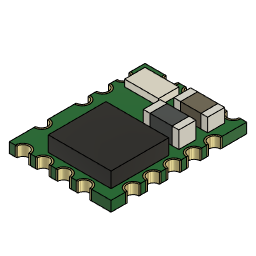
BLE-RN4871U v1 (Autodesk Fusion 360 design; units mm, degrees)
Autodesk Fusion 360 part; units mm, degrees
sketch "Sketch1" plane through (0, 0, 0) normal (0, 0, 1) x (1, 0, 0)
  arc A0 (6, 6.55) -> (6, 5.65) centre (6, 6.1) ccw
  arc A1 (6, 6.45) -> (6, 5.75) centre (6, 6.1) ccw
  arc A2 (6, 5.35) -> (6, 4.45) centre (6, 4.9) ccw
  arc A3 (6, 5.25) -> (6, 4.55) centre (6, 4.9) ccw
  arc A4 (6, 4.15) -> (6, 3.25) centre (6, 3.7) ccw
  arc A5 (6, 4.05) -> (6, 3.35) centre (6, 3.7) ccw
  arc A6 (6, 2.85) -> (6, 2.15) centre (6, 2.5) ccw
  arc A7 (6, 2.95) -> (6, 2.05) centre (6, 2.5) ccw
  arc A8 (6, 1.75) -> (6, 0.85) centre (6, 1.3) ccw
  arc A9 (6, 1.65) -> (6, 0.95) centre (6, 1.3) ccw
  arc A10 (4.85, 0) -> (3.95, 0) centre (4.4, 0) ccw
  arc A11 (4.75, 0) -> (4.05, 0) centre (4.4, 0) ccw
  arc A12 (3.65, 0) -> (2.75, 0) centre (3.2, 0) ccw
  arc A13 (3.55, 0) -> (2.85, 0) centre (3.2, 0) ccw
  arc A14 (2.45, 0) -> (1.55, 0) centre (2, 0) ccw
  arc A15 (2.35, 0) -> (1.65, 0) centre (2, 0) ccw
  arc A16 (1.25, 0) -> (0.35, 0) centre (0.8, 0) ccw
  arc A17 (1.15, 0) -> (0.45, 0) centre (0.8, 0) ccw
  arc A18 (0, 1.45) -> (0, 2.35) centre (0, 1.9) ccw
  arc A19 (0, 1.55) -> (0, 2.25) centre (0, 1.9) ccw
  arc A20 (0, 3.85) -> (0, 4.75) centre (0, 4.3) ccw
  arc A21 (0, 3.95) -> (0, 4.65) centre (0, 4.3) ccw
  arc A22 (0, 5.05) -> (0, 5.95) centre (0, 5.5) ccw
  arc A23 (0, 5.15) -> (0, 5.85) centre (0, 5.5) ccw
  arc A24 (0, 6.25) -> (0, 7.15) centre (0, 6.7) ccw
  arc A25 (0, 6.35) -> (0, 7.05) centre (0, 6.7) ccw
  arc A26 (1.15, 8) -> (2.05, 8) centre (1.6, 8) ccw
  arc A27 (1.25, 8) -> (1.95, 8) centre (1.6, 8) ccw
  arc A28 (2.35, 8) -> (3.25, 8) centre (2.8, 8) ccw
  arc A29 (2.45, 8) -> (3.15, 8) centre (2.8, 8) ccw
  arc A30 (3.65, 8) -> (4.35, 8) centre (4, 8) ccw
  arc A31 (3.55, 8) -> (4.45, 8) centre (4, 8) ccw
  arc A32 (4.75, 8) -> (5.65, 8) centre (5.2, 8) ccw
  arc A33 (4.85, 8) -> (5.55, 8) centre (5.2, 8) ccw
  line L0 (0, 1.55) -> (0, 0)
  line L1 (0, 3.95) -> (0, 2.25)
  line L2 (0, 5.15) -> (0, 4.65)
  line L3 (0, 8) -> (0, 7.05)
  line L4 (0, 6.35) -> (0, 5.85)
  line L5 (1.25, 8) -> (0, 8)
  line L6 (2.45, 8) -> (1.95, 8)
  line L7 (3.65, 8) -> (3.15, 8)
  line L8 (6, 8) -> (5.55, 8)
  line L9 (4.85, 8) -> (4.35, 8)
  line L10 (6, 6.45) -> (6, 8)
  line L11 (6, 5.25) -> (6, 5.75)
  line L12 (6, 4.05) -> (6, 4.55)
  line L13 (0, 0) -> (0.45, 0)
  line L14 (1.15, 0) -> (1.65, 0)
  line L15 (2.35, 0) -> (2.85, 0)
  line L16 (3.55, 0) -> (3.95, 0)
  line L17 (4.75, 0) -> (6, 0)
  line L18 (6, 0) -> (6, 0.95)
  line L19 (6, 1.65) -> (6, 2.15)
  line L20 (6, 2.85) -> (6, 3.35)
  line L21 (1.7, 4) -> (5.4, 4)
  line L22 (5.4, 4) -> (5.4, 0.6)
  line L23 (5.4, 0.6) -> (1.7, 0.6)
  line L24 (1.7, 0.6) -> (1.7, 4)
  line L25 (4.05, 0) -> (3.95, 0)
  line L26 (0.6, 7.4) -> (2.6, 7.4)
  line L27 (2.6, 7.4) -> (2.6, 6.2)
  line L28 (2.6, 6.2) -> (0.6, 6.2)
  line L29 (0.6, 6.2) -> (0.6, 7.4)
  line L30 (5.4, 4.6) -> (3.3, 4.6)
  line L31 (3.3, 4.6) -> (3.3, 5.6)
  line L32 (3.3, 5.6) -> (5.4, 5.6)
  line L33 (5.4, 5.6) -> (5.4, 4.6)
  line L34 (5.4, 6.3) -> (3.4, 6.3)
  line L35 (3.4, 6.3) -> (3.4, 7.3)
  line L36 (3.4, 7.3) -> (5.4, 7.3)
  line L37 (5.4, 7.3) -> (5.4, 6.3)
  line L38 (3.8, 6.3) -> (3.8, 7.3)
  line L39 (5, 6.3) -> (5, 7.3)
  line L40 (3.7, 5.6) -> (3.7, 4.6)
  line L41 (5, 5.6) -> (5, 4.6)
  constraint horizontal L13
  constraint vertical L18
  constraint horizontal L8
  constraint vertical L3
  constraint coincident L0.end L13.start
  constraint concentric A16 A17
  constraint concentric A14 A15
  constraint concentric A12 A13
  constraint concentric A10 A11
  constraint concentric A18 A19
  constraint concentric A20 A21
  constraint concentric A22 A23
  constraint concentric A24 A25
  constraint concentric A8 A9
  constraint concentric A6 A7
  constraint concentric A4 A5
  constraint concentric A2 A3
  constraint concentric A0 A1
  constraint concentric A26 A27
  constraint concentric A28 A29
  constraint concentric A30 A31
  constraint concentric A32 A33
  constraint coincident A0.end L18
  constraint coincident A0.start L18
  constraint coincident A1.start L18
  constraint coincident A2.end L18
  constraint coincident A2.start L18
  constraint coincident A3.start L18
  constraint coincident A4.end L18
  constraint coincident A4.start L18
  constraint coincident A5.start L18
  constraint coincident A6.end L18
  constraint coincident A6.start L18
  constraint coincident A7.end L18
  constraint coincident A7.start L18
  constraint coincident A8.end L18
  constraint coincident A8.start L18
  constraint coincident A9.start L18
  constraint coincident A10.end L13
  constraint coincident A10.start L13
  constraint coincident A11.end L13
  constraint coincident A11.start L13
  constraint coincident A12.end L13
  constraint coincident A12.start L13
  constraint coincident A13.end L13
  constraint coincident A13.start L13
  constraint coincident A14.end L13
  constraint coincident A14.start L13
  constraint coincident A15.end L13
  constraint coincident A15.start L13
  constraint coincident A16.end L13
  constraint coincident A16.start L13
  constraint coincident A17.start L13
  constraint coincident A18.end L3
  constraint coincident A18.start L3
  constraint coincident A19.start L3
  constraint coincident A20.end L3
  constraint coincident A20.start L3
  constraint coincident A21.start L3
  constraint coincident A22.end L3
  constraint coincident A22.start L3
  constraint coincident A23.start L3
  constraint coincident A24.end L3
  constraint coincident A24.start L3
  constraint coincident A25.start L3
  constraint coincident A26.end L8
  constraint coincident A26.start L8
  constraint coincident A27.start L8
  constraint coincident A28.end L8
  constraint coincident A28.start L8
  constraint coincident A29.start L8
  constraint coincident A30.start L8
  constraint coincident A31.end L8
  constraint coincident A31.start L8
  constraint coincident A32.end L8
  constraint coincident A32.start L8
  constraint coincident A33.start L8
  constraint collinear L0 L3
  constraint collinear L1 L3
  constraint collinear L2 L3
  constraint collinear L3 L4
  constraint collinear L5 L8
  constraint collinear L6 L8
  constraint collinear L7 L8
  constraint collinear L8 L9
  constraint collinear L10 L18
  constraint collinear L11 L18
  constraint collinear L12 L18
  constraint collinear L13 L14
  constraint collinear L14 L15
  constraint collinear L15 L16
  constraint collinear L16 L17
  constraint collinear L18 L19
  constraint collinear L19 L20
  constraint horizontal L21
  constraint vertical L22
  constraint horizontal L23
  constraint vertical L24
  constraint horizontal L26
  constraint vertical L27
  constraint horizontal L28
  constraint vertical L29
  constraint horizontal L32
  constraint vertical L33
  constraint horizontal L30
  constraint vertical L31
  constraint horizontal L36
  constraint vertical L37
  constraint horizontal L34
  constraint vertical L35
  constraint coincident L36 L38.end
  constraint perpendicular L36 L38
  constraint coincident L36 L39.end
  constraint perpendicular L36 L39
  constraint coincident L30 L40.end
  constraint perpendicular L30 L40
  constraint coincident L30 L41.end
  constraint perpendicular L30 L41
  constraint coincident L32 L40.start
  constraint coincident L34 L38.start
  constraint coincident L34 L39.start
  constraint coincident L32 L41.start
extrude "Extrude1" add sketch "Sketch1" along normal blind 0.6 contours A0 A2 A4 A7 A8 A10 A12 A14 A16 A18 A20 A22 A24 A26 A28 A31 A32 L0 L1 L2 L3 L4 L5 L6 L7 L8 L9 L10 L11 L12 L13 L14 L15 L16 L17 L18 L19 L20 | L21 L22 L23 L24 | L26 L27 L28 L29 | L30 L32 L33 L41 | L30 L32 L40 L41 | L30 L31 L32 L40 | L34 L36 L37 L39 | L34 L36 L38 L39 | L34 L35 L36 L38 makes body 1
extrude "Extrude2" add sketch "Sketch1" along normal blind 0.6 separate body contours A0 A1 L10 L11 | A2 A3 L11 L12 | A32 A33 L8 L9 | A4 A5 L12 L20 | A30 A31 L7 L9 | A6 A7 L19 L20 | A28 A29 L6 L7 | A8 A9 L18 L19 | A26 A27 L5 L6 | A10 A11 L17 L25 | A24 A25 L3 L4 | A12 A13 L15 L16 | A22 A23 L2 L4 | A14 A15 L14 L15 | A20 A21 L1 L2 | A16 A17 L13 L14 | A18 A19 L0 L1 makes body 2 at (1.8149, 0.4102, 0.2) makes body 3 at (5.8252, 4.1147, 0.4) makes body 4 at (4.2978, 7.6626, 0.2) makes body 5 at (0.4332, 5.3781, 0.4) makes body 6 at (0.4465, 6.644, 0.4) makes body 7 at (5.5447, 7.7107, 0.4) makes body 8 at (5.9108, 2.0589, 0.4) makes body 9 at (0.416, 0.2346, 0.4) makes body 10 at (3.3219, 0.4332, 0.4) makes body 11 at (5.5734, 5.0433, 0.4) makes body 12 at (3.1447, 7.7107, 0.4) makes body 13 at (0.4465, 4.244, 0.4) makes body 14 at (1.9447, 7.7107, 0.4) makes body 15 at (5.5734, 6.2433, 0.4) makes body 16 at (5.8252, 1.7147, 0.4) makes body 17 at (0.0224, 2.3494, 0.4) makes body 18 at (4.6978, 0.3374, 0.4)
extrude "Extrude3" add sketch "Sketch1" along normal blind 0.6 and the other way blind -1.5 separate body contours L21 L22 L23 L24 makes body 19
extrude "Extrude4" add sketch "Sketch1" along normal blind 1 and the other way blind -0.6 separate body contours L26 L27 L28 L29 makes body 20
extrude "Extrude5" add sketch "Sketch1" along normal blind 1.6 and the other way blind -0.6 separate body contours L30 L32 L33 L41 | L30 L31 L32 L40 makes body 21 at (5, 5.2667, 0.9333) makes body 22 at (3.3, 4.9333, 0.9333)
extrude "Extrude6" add sketch "Sketch1" along normal blind 1.4 and the other way blind -0.6 separate body contours L34 L36 L37 L39 | L34 L35 L36 L38 makes body 23 at (5, 6.6333, 0.8667) makes body 24 at (3.4, 6.6333, 0.8667)
extrude "Extrude7" add sketch "Sketch1" along normal blind 1.6 and the other way blind -0.6 separate body contours L30 L32 L40 L41 makes body 25
extrude "Extrude8" add sketch "Sketch1" along normal blind 1.4 and the other way blind -0.6 separate body contours L34 L36 L38 L39 makes body 26
equation "d37 = 0.6 mm + 0.4 mm"
